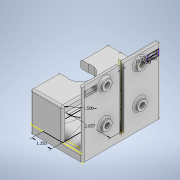
# Autodesk Inventor part: CatchlessCatchHolder
Saved by Autodesk Inventor 2020 (Build 240168000, 168)
## iProperties
Created: 2021-07-14
Part Number: CatchlessCatchHolder
Material: Generic
Document SubType Name: Modeling
Designer: pab2
Density: 1 g/cm^3
Appearance: Default
Author: pab2
Autodesk Inventor part; units mm, degrees
ref_plane "YZ Plane" through (0, 0, 0) normal (1, 0, 0) x (0, 1, 0)
ref_plane "XZ Plane" through (0, 0, 0) normal (0, 1, 0) x (-1, 0, 0)
ref_plane "XY Plane" through (0, 0, 0) normal (0, 0, 1) x (1, 0, 0)
sketch "Sketch1" plane through (0, 0, 0) normal (0, 1, 0) x (-1, 0, 0)
  line L0 (0, 0) -> (85.48, 0)
  line L1 (85.48, 0) -> (85.48, -127.76)
  line L2 (85.48, -127.76) -> (0, -127.76)
  line L3 (0, -127.76) -> (0, 0)
  line L4 (0, 0) -> (7.0711, -7.0711)
  line L5 (0, 0) -> (10, 0) construction
  circle A0 centre (7.0711, -7.0711) radius 4.7625
  dimension "d0" = 85.48
  dimension "d1" = 127.76
  dimension "offsetDiag" = 10
  dimension "d3" = 45
  dimension "d4" = 9.525
  constraints: 12 end point, 2 horizontal, 2 parallel, 1 centre point, 1 coincident, 1 equal length, 1 perpendicular
  measures "d0" distance of L1.end L2.end
  measures "d1" distance of L0.end L1.end
  measures "offsetDiag" distance of L0.start L4.end
  measures "d3" angle of L4 L5
  measures "d4" diameter of A0
extrude "Extrusion1" add sketch "Sketch1" along normal blind 12.7 contours L0 L1 L2 L3 | A0
sketch "Sketch3" plane through (0, 12.7, 0) normal (0, 1, 0) x (1, 0, 0)
  line L0 (0, 0) -> (0, 127.76) projected
  line L1 (0, 63.88) -> (-72.5, 63.88)
  line L2 (-140, 121.63) -> (-5, 121.63)
  line L3 (-5, 121.63) -> (-5, 6.13)
  line L4 (-5, 6.13) -> (-140, 6.13)
  line L5 (-140, 6.13) -> (-140, 121.63)
  line L6 (-140, 121.63) -> (-5, 6.13) construction
  line L7 (-5, 121.63) -> (-140, 6.13) construction
  dimension "d23" = 72.5
  dimension "d24" = 135
  dimension "d25" = 115.5
  constraints: 14 end point, 3 midpoint, 2 horizontal, 2 parallel, 1 perpendicular
  measures "d23" distance of L1.start L1.end
  measures "d24" distance of L3.end L4.end
  measures "d25" distance of L2.end L3.end
extrude "Extrusion2" cut sketch "Sketch3" against normal blind 2.54
sketch "Sketch4" plane through (0, 12.7, 0) normal (0, 1, 0) x (1, 0, 0)
  line L0 (-5, 121.63) -> (-5, 6.13) projected
  line L1 (5, 67.055) -> (-5, 67.055)
  line L2 (-5, 67.055) -> (-5, 60.705)
  line L3 (-5, 60.705) -> (5, 60.705)
  line L4 (5, 60.705) -> (5, 67.055)
  line L5 (0, 0) -> (0, 127.76) projected
  line L6 (5, 67.055) -> (-5, 60.705) construction
  line L7 (-5, 67.055) -> (5, 60.705) construction
  point P0 (0, 63.88)
  point P1 (0, 60.705)
  point P2 (0, 67.055)
  dimension "d28" = 6.35
  constraints: 12 end point, 3 midpoint, 2 parallel, 1 horizontal, 1 perpendicular, 1 point on line
  measures "d28" distance of L2.end L1.end
extrude "Extrusion3" cut sketch "Sketch4" against normal blind 2.54 contours L1 L5 L3 L0
sketch "Sketch5" plane through (0, 12.7, 0) normal (0, 1, 0) x (1, 0, 0)
  line L0 (0, 67.055) -> (0, 60.705) projected
  line L1 (0, 63.88) -> (-67.5, 63.88)
  circle A0 centre (-67.5, 63.88) radius 19.05
  line L2 (-85.48, 0) -> (0, 0) projected
  line L3 (-64.325, 127.76) -> (-32.575, 127.76)
  line L4 (-32.575, 127.76) -> (-32.575, 0)
  line L5 (-32.575, 0) -> (-64.325, 0)
  line L6 (-64.325, 0) -> (-64.325, 127.76)
  line L7 (-64.325, 127.76) -> (-32.575, 0) construction
  line L8 (-32.575, 127.76) -> (-64.325, 0) construction
  line L9 (-85.48, 121.63) -> (-5, 121.63) projected
  line L10 (-62.8016, 121.63) -> (-32.575, 121.63)
  line L11 (-32.575, 121.63) -> (-32.575, 127.76)
  line L12 (-32.575, 127.76) -> (-62.8016, 127.76)
  line L13 (-62.8016, 127.76) -> (-62.8016, 121.63)
  line L14 (-5, 6.13) -> (-85.48, 6.13) projected
  line L15 (-64.325, 0) -> (-32.575, 0)
  line L16 (-32.575, 0) -> (-32.575, 6.13)
  line L17 (-32.575, 6.13) -> (-64.325, 6.13)
  line L18 (-64.325, 6.13) -> (-64.325, 0)
  point P0 (-48.45, 63.88)
  point P1 (-64.325, 6.13)
  point P2 (-32.575, 121.63)
  dimension "d32" = 38.1
  dimension "d31" = 67.5
  dimension "d33" = 31.75
  constraints: 30 end point, 6 parallel, 6 point on line, 4 horizontal, 3 midpoint, 3 perpendicular, 1 coincident, 1 horizontal alignment, 2 other
  measures "d31" distance of L1.start L1.end
  measures "d33" distance of L4.end L5.end
extrude "Extrusion4" add sketch "Sketch5" along normal blind 50 contours L9 L13 L3 L4 | L4 L2 L6 L14
sketch "Sketch6" plane through (-85.48, 10.16, -121.63) normal (0, 0, 1) x (1, 0, 0)
  line L0 (52.905, 2.54) -> (52.905, 52.54) projected
  line L1 (21.155, 52.54) -> (52.905, 52.54)
  line L2 (52.905, 52.54) -> (52.905, 39.84)
  line L3 (52.905, 39.84) -> (21.155, 39.84)
  line L4 (21.155, 39.84) -> (21.155, 52.54)
  line L5 (22.6784, 2.54) -> (22.6784, 52.54) projected
  line L6 (22.6784, 52.54) -> (52.905, 52.54)
  line L7 (52.905, 52.54) -> (52.905, 39.84)
  line L8 (52.905, 39.84) -> (22.6784, 39.84)
  line L9 (22.6784, 39.84) -> (22.6784, 52.54)
  point P0 (85.48, -10.16)
  point P1 (22.6784, 39.84)
  dimension "d36" = 12.7
  constraints: 16 end point, 4 parallel, 2 horizontal, 2 perpendicular, 1 point on line
  measures "d36" distance of L1.end L2.end
extrude "Extrusion5" add sketch "Sketch6" along normal up to surface (121.63 mm away) contours L3 L5 L1 L0
sketch "Sketch7" plane through (0, 62.7, 0) normal (0, 1, 0) x (1, 0, 0)
  line L0 (-32.575, 121.63) -> (-32.575, 6.13) projected
  line L1 (-32.575, 63.88) -> (-67.3875, 63.88)
  circle A0 centre (-67.3875, 63.88) radius 19.05
  point P0 (0, 0)
  dimension "d39" = 38.1
  constraints: 2 end point, 1 centre point, 1 coincident, 1 horizontal, 1 midpoint
  measures "d39" diameter of A0
extrude "Extrusion6" cut sketch "Sketch7" against normal blind 25.4
sketch "Sketch8" plane through (-32.575, 12.7, 0) normal (1, 0, 0) x (0, 0, -1)
  line L0 (0, 50) -> (127.76, 50) projected
  line L1 (63.88, 50) -> (63.88, 37.3)
  line L2 (121.63, 37.3) -> (6.13, 37.3) projected
  line L3 (63.88, 43.65) -> (76.58, 43.65)
  line L4 (82.3698, 37.3) -> (82.3698, 50) projected
  line L5 (63.88, 43.65) -> (76.58, 43.65) construction
  line L6 (63.88, 43.65) -> (51.18, 43.65)
  point P0 (0, -12.7)
  dimension "d42" = 12.7
  dimension "d43" = 0
  dimension "d44" = 12.7
  constraints: 8 end point, 3 midpoint, 2 horizontal, 1 collinear, 1 perpendicular
  measures "d42" distance of L3.start L3.end
  measures "d43" distance between parallel lines of L3 L5
  measures "d44" distance of L3.start L6.end
hole "Hole2" at (-32.575, 56.35, -51.18) at (-32.575, 56.35, -76.58) direction (-1, 0, 0) diameter 5.1054 depth 35 clearance for "Flat Head Machine Screw (82)" size "#10" standard "Ansi Unified Screw Threads"
sketch "Sketch9" plane through (0, 12.7, 0) normal (0, 1, 0) x (1, 0, 0)
  line L0 (0, 127.76) -> (-85.48, 127.76) projected
  line L1 (-85.48, 121.63) -> (-5, 121.63) projected
  line L2 (-85.48, 127.76) -> (-62.8343, 127.76)
  line L3 (-62.8343, 127.76) -> (-62.8343, 121.63)
  line L4 (-62.8343, 121.63) -> (-85.48, 121.63)
  line L5 (-85.48, 121.63) -> (-85.48, 127.76)
  line L6 (-5, 6.13) -> (-85.48, 6.13) projected
  line L7 (-85.48, 0) -> (0, 0) projected
  line L8 (-85.48, 6.13) -> (-64.2002, 6.13)
  line L9 (-64.2002, 6.13) -> (-64.2002, 0)
  line L10 (-64.2002, 0) -> (-85.48, 0)
  line L11 (-85.48, 0) -> (-85.48, 6.13)
  constraints: 16 end point, 4 parallel, 2 horizontal, 2 perpendicular, 2 point on line
extrude "Extrusion7" add sketch "Sketch9" along normal blind 50
sketch "Sketch10" plane through (-62.8016, 12.7, -127.76) normal (-1, 0, 0) x (0, 0, 1)
  line L0 (6.13, -2.54) -> (6.13, 50) projected
  line L1 (127.76, 50) -> (0, 50) projected
  line L2 (6.13, 37.3853) -> (45.4987, 37.3853)
  line L3 (45.4987, 37.3853) -> (45.4987, 50)
  line L4 (45.4987, 50) -> (6.13, 50)
  line L5 (6.13, 50) -> (6.13, 37.3853)
  line L6 (82.3698, 50) -> (82.3698, 37.3) projected
  line L7 (121.63, 50) -> (127.76, 50) projected
  line L8 (82.3698, 37.3) -> (127.76, 37.3)
  line L9 (127.76, 37.3) -> (127.76, 50)
  line L10 (127.76, 50) -> (82.3698, 50)
  line L11 (82.3698, 50) -> (82.3698, 37.3)
  point P0 (127.76, -12.7)
  constraints: 16 end point, 4 parallel, 2 horizontal, 2 perpendicular, 2 point on line
extrude "Extrusion8" add sketch "Sketch10" along normal up to surface (22.6784 mm away)
sketch "Sketch11" plane through (0, 62.7, 0) normal (0, 1, 0) x (1, 0, 0)
  line L0 (-32.575, 121.63) -> (-32.575, 6.13) projected
  line L1 (-32.575, 63.88) -> (-67.3716, 63.88)
  circle A0 centre (-67.3716, 63.88) radius 19.0354
  point P0 (0, 0)
  constraints: 2 end point, 1 centre point, 1 coincident, 1 horizontal, 1 midpoint
extrude "Extrusion9" cut sketch "Sketch11" against normal blind 38.1
sketch "Sketch12" plane through (0, 12.7, 0) normal (0, 1, 0) x (1, 0, 0)
  line L0 (-5, 67.055) -> (0, 67.055) projected
  line L1 (0, 127.76) -> (-32.575, 127.76) projected
  line L2 (0, 67.055) -> (-5.3059, 67.055)
  line L3 (-5.3059, 67.055) -> (-5.3059, 127.76)
  line L4 (-5.3059, 127.76) -> (0, 127.76)
  line L5 (0, 127.76) -> (0, 67.055)
  line L6 (-5, 60.705) -> (-5, 6.13) projected
  line L7 (-5, 60.705) -> (0, 60.705)
  line L8 (0, 60.705) -> (0, 0)
  line L9 (0, 0) -> (-5, 0)
  line L10 (-5, 0) -> (-5, 60.705)
  constraints: 16 end point, 4 parallel, 2 horizontal, 2 perpendicular, 1 point on line
extrude "Extrusion10" add sketch "Sketch12" along normal blind 95.25
sketch "Sketch13" plane through (0, 0, 0) normal (1, 0, 0) x (0, 0, -1)
  line L0 (6.13, 10.16) -> (121.63, 10.16) projected
  line L1 (63.88, 10.16) -> (63.88, 0)
  line L2 (127.76, 0) -> (0, 0) projected
  line L3 (63.88, 0) -> (92.455, 0)
  line L4 (92.455, 0) -> (92.455, 37.846)
  line L5 (92.455, 37.846) -> (35.305, 37.846)
  line L6 (35.305, 37.846) -> (35.305, 94.996)
  line L7 (35.305, 94.996) -> (92.455, 94.996)
  dimension "d60" = 28.575
  dimension "d61" = 37.846
  dimension "d62" = 57.15
  dimension "d63" = 57.15
  dimension "d64" = 90
  dimension "d65" = 57.15
  dimension "d66" = 90
  constraints: 12 end point, 4 perpendicular, 2 midpoint, 1 point on line
  measures "d60" distance of L1.end L3.end
  measures "d61" distance of L3.end L4.end
  measures "d62" distance of L4.end L5.end
  measures "d63" distance of L5.end L6.end
  measures "d64" angle of L5 L6
  measures "d65" distance of L6.end L7.end
  measures "d66" angle of L6 L7
hole "Hole3" at (0, 37.846, -35.305) at (0, 94.996, -35.305) at (0, 94.996, -92.455) at (0, 37.846, -92.455) direction (-1, 0, 0) diameter 8.4328 end through all
sketch "Sketch14" plane through (-85.48, 0, 0) normal (0, 0, 1) x (1, 0, 0)
  line L0 (80.1741, 107.95) -> (85.48, 107.95) projected
  circle A0 centre (82.827, 107.95) radius 2.653
  line L1 (85.48, 0) -> (85.48, 107.95) projected
  constraints: 1 centre point, 1 midpoint, 1 tangent
extrude "Extrusion11" cut sketch "Sketch14" against normal through all
sketch "Sketch15" plane through (0, 0, 0) normal (1, 0, 0) x (0, 0, -1)
  circle A0 centre (35.305, 94.996) radius 4.2164 projected
  circle A1 centre (35.305, 94.996) radius 7.9375
  circle A2 centre (92.455, 94.996) radius 4.2164 projected
  circle A3 centre (92.455, 94.996) radius 7.9375
  circle A4 centre (92.455, 37.846) radius 4.2164 projected
  circle A5 centre (92.455, 37.846) radius 7.9375
  circle A6 centre (35.305, 37.846) radius 4.2164 projected
  circle A7 centre (35.305, 37.846) radius 7.9375
  circle A8 centre (35.305, 94.996) radius 4.2164
  circle A9 centre (92.455, 94.996) radius 4.2164
  circle A10 centre (35.305, 37.846) radius 4.2164 projected
  circle A11 centre (35.305, 37.846) radius 2.1082
  circle A12 centre (92.455, 37.846) radius 4.2164
  point P0 (0, 0)
  dimension "d76" = 15.875
  dimension "d77" = 15.875
  dimension "d78" = 15.875
  dimension "d79" = 15.875
  constraints: 8 centre point, 8 coincident, 3 concentric
  measures "d76" diameter of A1
  measures "d77" diameter of A3
  measures "d78" diameter of A5
  measures "d79" diameter of A7
extrude "Extrusion12" add sketch "Sketch15" along normal blind 5.08 contours A1 | A3 | A5 | A7
sketch "Sketch16" plane through (-5, 12.7, -6.13) normal (-1, 0, 0) x (0, 0, 1)
  circle A0 centre (-86.325, 82.296) radius 4.2164 projected
  line L0 (-86.325, 82.296) -> (-86.325, 87.63)
  line L1 (-60.925, 92.597) -> (-121.63, 92.597) projected
  line L2 (-86.325, 87.63) -> (-60.925, 87.63)
  line L3 (-60.925, 95.25) -> (-60.925, -2.54) projected
  line L4 (-86.325, 87.63) -> (-57.75, 87.63)
  line L5 (-57.75, 87.63) -> (-62.449, 87.63)
  line L6 (-62.449, 87.63) -> (-53.051, 87.63)
  point P0 (6.13, -12.7)
  dimension "d64" = 90
  dimension "d65" = 57.15
  dimension "d66" = 90
  dimension "d82" = 5.334
  dimension "d83" = 28.575
  dimension "d84" = 4.699
  dimension "d85" = 9.398
  constraints: 10 end point, 4 point on line, 1 horizontal, 1 perpendicular
  measures "d82" distance of L0.start L0.end
  measures "d83" distance of L0.end L4.end
  measures "d84" distance of L4.end L5.end
  measures "d85" distance of L5.end L6.end
hole "Hole4" at (-5, 100.33, -59.181) at (-5, 100.33, -68.579) direction (-1, 0, 0) diameter 2.286 end through all both
sketch "Sketch17" plane through (0, 0, 0) normal (1, 0, 0) x (0, 0, -1)
  circle A0 centre (92.455, 94.996) radius 4.2164 projected
  line L0 (92.455, 94.996) -> (101.98, 94.996)
  line L1 (92.455, 94.996) -> (101.98, 94.996) construction
  line L2 (101.98, 94.996) -> (108.33, 94.996)
  line L3 (108.33, 94.996) -> (121.03, 94.996)
  line L4 (124.205, 99.7585) -> (105.155, 99.7585)
  line L5 (105.155, 99.7585) -> (105.155, 90.2335)
  line L6 (105.155, 90.2335) -> (124.205, 90.2335)
  line L7 (124.205, 90.2335) -> (124.205, 99.7585)
  line L8 (124.205, 99.7585) -> (105.155, 90.2335) construction
  line L9 (105.155, 99.7585) -> (124.205, 90.2335) construction
  point P0 (0, 0)
  point P1 (114.68, 94.996)
  dimension "d93" = 9.525
  dimension "d94" = 0
  dimension "d95" = 6.35
  dimension "d96" = 12.7
  dimension "d97" = 9.525
  constraints: 20 end point, 3 horizontal, 3 midpoint, 2 parallel, 2 point on line, 1 collinear, 1 perpendicular
  measures "d93" distance of L0.start L0.end
  measures "d94" distance between parallel lines of L0 L1
  measures "d95" distance of L0.end L2.end
  measures "d96" distance of L2.end L3.end
  measures "d97" distance of L5.end L4.end
extrude "Extrusion13" cut sketch "Sketch17" against normal blind 3.175 contours L7 L6 L5 L4
hole "Hole5" at (0, 94.996, -121.03) at (0, 94.996, -108.33) direction (-1, 0, 0) diameter 3.2766 end through all clearance for "Flat Head Machine Screw (82)" size "#4" standard "Ansi Unified Screw Threads"
ref_plane "Work Plane1" through (0, 10.16, -63.88) normal (0, 0, -1) x (-1, 0, 0)
mirror "Mirror1" about plane through (0, 10.16, -63.88) normal (0, 0, -1) of "Extrusion13", "Hole5"
fillet "Fillet1" radius 3.175 27 edges at (-32.575, 37.7, 0) (-59.0275, 62.7, 0) (-85.48, 62.7, -22.6951) (-85.48, 62.7, -105.0106) (-74.1571, 62.7, -127.76) (-47.6883, 62.7, -127.76) (-32.575, 62.7, -63.88) (-85.48, 50.0853, -101.9456) (-85.48, 50, -25.7601) (-85.48, 30.1226, -121.63) (-85.48, 30.08, -6.13) (-32.575, 31.35, -121.63) (-32.575, 50, -63.88) (-18.9405, 12.7, -127.76) (-18.7875, 12.7, 0) (-5, 59.7066, 0) (0, 53.975, 0) (0, 53.975, -127.76) (-5.3059, 60.325, -127.76) (-32.575, 37.7, -127.76) (-32.575, 31.35, -6.13) (-85.48, 31.35, 0) (-85.48, 31.35, -127.76) (0, 94.996, -27.3675) (0, 94.996, -84.5175) (0, 37.846, -84.5175) (0, 37.846, -27.3675)
body "Solid1"
